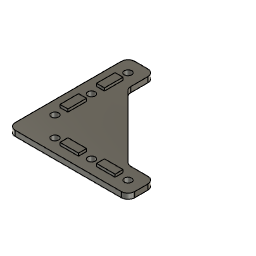
Corner Brace (Autodesk Fusion 360 design; units mm, degrees)
Autodesk Fusion 360 part; units mm, degrees
sketch "Sketch1" plane through (0, 0, 0) normal (0, 0, 1) x (1, 0, 0)
  line L0 (0, 0) -> (0, 90)
  line L1 (0, 0) -> (90, 0)
  line L2 (0, 90) -> (20, 90)
  line L3 (90, 0) -> (90, 20)
  line L4 (90, 20) -> (70, 20)
  line L5 (20, 90) -> (20, 70)
  line L6 (20, 70) -> (70, 20)
  line L7 (10, 90) -> (10, 0) construction
  line L8 (90, 10) -> (0, 10) construction
  circle A0 centre (80, 10) radius 2.75
  circle A1 centre (25, 10) radius 2.75
  circle A2 centre (52.5, 10) radius 2.75
  line L9 (0, 0) -> (79.8876, 79.8876) construction
  line L10 (0, 0) -> (112.9781, 0) construction
  line L11 (25, 10) -> (52.5, 10) construction
  line L12 (52.5, 10) -> (80, 10) construction
  line L13 (45.75, 7) -> (31.75, 7)
  line L14 (31.75, 7) -> (31.75, 13)
  line L15 (31.75, 13) -> (45.75, 13)
  line L16 (45.75, 13) -> (45.75, 7)
  line L17 (45.75, 7) -> (31.75, 13) construction
  line L18 (31.75, 7) -> (45.75, 13) construction
  line L19 (73.25, 7) -> (59.25, 7)
  line L20 (59.25, 7) -> (59.25, 13)
  line L21 (59.25, 13) -> (73.25, 13)
  line L22 (73.25, 13) -> (73.25, 7)
  line L23 (73.25, 7) -> (59.25, 13) construction
  line L24 (59.25, 7) -> (73.25, 13) construction
  circle A3 centre (10, 25) radius 2.75
  line L25 (7, 31.75) -> (13, 31.75)
  line L26 (13, 31.75) -> (13, 45.75)
  line L27 (7, 45.75) -> (7, 31.75)
  line L28 (13, 45.75) -> (7, 45.75)
  line L29 (7, 59.25) -> (13, 59.25)
  line L30 (13, 59.25) -> (13, 73.25)
  line L31 (13, 73.25) -> (7, 73.25)
  line L32 (7, 73.25) -> (7, 59.25)
  circle A4 centre (10, 80) radius 2.75
  circle A5 centre (10, 52.5) radius 2.75
  point P0 (38.75, 10)
  point P1 (66.25, 10)
  dimension "d1" = 90
  dimension "d2" = 90
  dimension "d3" = 20
  dimension "d4" = 20
  dimension "d5" = 20
  dimension "d6" = 20
  dimension "d7" = 5.5
  dimension "d8" = 5.5
  dimension "d9" = 10
  dimension "d10" = 65
  dimension "d11" = 5.5
  dimension "d12" = 37.5
  dimension "d13" = 45
  dimension "d14" = 14
  dimension "d15" = 6
  dimension "d16" = 14
  dimension "d17" = 6
  constraint coincident L0.start L1.start
  constraint vertical L0
  constraint perpendicular L0 L1
  constraint perpendicular L0 L2
  constraint perpendicular L1 L3
  constraint perpendicular L3 L4
  constraint perpendicular L2 L5
  constraint midpoint L2 L7.start
  constraint coincident L1 L7.end
  constraint perpendicular L1 L7
  constraint midpoint L3 L8.start
  constraint coincident L0 L8.end
  constraint perpendicular L0 L8
  constraint coincident L8 A0.centre
  constraint coincident L8 A1.centre
  constraint coincident L8 A2.centre
  constraint horizontal L10
  constraint coincident A1.centre L11.start
  constraint coincident A2.centre L11.end
  constraint coincident A0.centre L12.end
  constraint horizontal L13
  constraint perpendicular L13 L14
  constraint parallel L13 L15
  constraint parallel L14 L16
  constraint coincident L17 P0
  constraint coincident L18 P0
  constraint midpoint L11 P0
  constraint horizontal L19
  constraint perpendicular L19 L20
  constraint parallel L19 L21
  constraint parallel L20 L22
  constraint coincident L23 P1
  constraint coincident L24 P1
  constraint midpoint L12 P1
  constraint symmetric A0 L9 A4
  constraint symmetric A1 L9 A3
  constraint symmetric A2 L9 A5
  constraint symmetric L9 L13.start L27.start
  constraint symmetric L9 L13.end L25.start
  constraint symmetric L9 L14.end L25.end
  constraint symmetric L9 L15.end L26.end
  constraint symmetric L9 L19.start L31.end
  constraint symmetric L9 L19.end L29.start
  constraint symmetric L9 L20.end L29.end
  constraint symmetric L9 L21.end L30.end
  measures "d1" distance of L0.start L0.end
  measures "d2" distance of L0.start L1.end
  measures "d3" distance of L0.end L2.end
  measures "d4" distance of L1.end L3.end
  measures "d5" distance of L3.end L4.end
  measures "d6" distance of L2.end L5.end
  measures "d7" diameter of A0
  measures "d8" diameter of A1
  measures "d9" distance of L8.start A0.centre
  measures "d10" distance of L3 A1.centre
  measures "d11" diameter of A2
  measures "d12" distance of L3 A2.centre
  measures "d13" angle of L9 L10
  measures "d14" distance of L14.end L15.end
  measures "d15" distance of L13.end L14.end
  measures "d16" distance of L20.end L21.end
  measures "d17" distance of L19.end L20.end
extrude "Extrude1" add sketch "Sketch1" along normal blind 4
extrude "Extrude3" add sketch "Sketch1" along normal blind 6 contours L13 L14 L15 L16 | L19 L20 L21 L22 | L25 L26 L27 L28 | L29 L30 L31 L32
sketch "Sketch2" plane through (0, 0, 4) normal (0, 0, 1) x (-1, 0, 0)
  circle A0 centre (-25, -10) radius 2.75
  circle A1 centre (-52.5, -10) radius 2.75
  circle A2 centre (-10, -80) radius 2.75
  circle A3 centre (-10, -25) radius 2.75
  circle A4 centre (-80, -10) radius 2.75
  circle A5 centre (-10, -52.5) radius 2.75
  line L0 (0, 0) -> (-90, 0)
  line L1 (-90, 0) -> (-90, -20)
  line L2 (-90, -20) -> (-70, -20)
  line L3 (-70, -20) -> (-20, -70)
  line L4 (-20, -70) -> (-20, -90)
  line L5 (-20, -90) -> (0, -90)
  line L6 (0, -90) -> (0, 0)
  line L7 (-20, -70) -> (-20, -20) construction
  line L8 (-20, -20) -> (-70, -20) construction
  line L9 (-20, -70) -> (-70, -20) construction
  line L10 (-23, -62.7574) -> (-62.7574, -23)
  line L11 (-23, -23) -> (-62.7574, -23)
  line L12 (-23, -62.7574) -> (-23, -23)
  line L13 (-7, -45.75) -> (-13, -45.75)
  line L14 (-13, -45.75) -> (-13, -31.75)
  line L15 (-13, -31.75) -> (-7, -31.75)
  line L16 (-7, -31.75) -> (-7, -45.75)
  line L17 (-59.25, -13) -> (-73.25, -13)
  line L18 (-73.25, -13) -> (-73.25, -7)
  line L19 (-73.25, -7) -> (-59.25, -7)
  line L20 (-59.25, -7) -> (-59.25, -13)
  line L21 (-7, -59.25) -> (-7, -73.25)
  line L22 (-7, -73.25) -> (-13, -73.25)
  line L23 (-13, -73.25) -> (-13, -59.25)
  line L24 (-13, -59.25) -> (-7, -59.25)
  line L25 (-31.75, -13) -> (-45.75, -13)
  line L26 (-45.75, -13) -> (-45.75, -7)
  line L27 (-45.75, -7) -> (-31.75, -7)
  line L28 (-31.75, -7) -> (-31.75, -13)
  dimension "d20" = 3
  constraint coincident L3.end L4.start
  constraint perpendicular L2 L7
  constraint coincident L2.end L3.start
  constraint perpendicular L7 L8
fillet "Fillet1" radius 5 7 edges at (0, 0, 2) (90, 0, 2) (90, 20, 2) (20, 70, 2) (70, 20, 2) (20, 90, 2) (0, 90, 2)
equation "d5 = d6"
